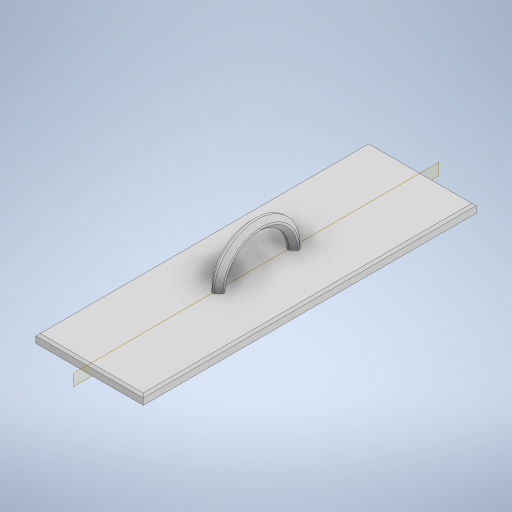
# Autodesk Inventor part: water lock
Saved by Autodesk Inventor 2023 (Build 270158000, 158)
## iProperties
Created: 2022-11-25
Part Number: water lock
Material: Generic
Document SubType Name: Sheet Metal
Designer: hp
Density: 1 g/cm^3
Sheet Metal Rule: Default_mm
Appearance: Default
Author: hp
Autodesk Inventor part; units mm, degrees
ref_plane "YZ Plane" through (0, 0, 0) normal (1, 0, 0) x (0, 1, 0)
ref_plane "XZ Plane" through (0, 0, 0) normal (0, 1, 0) x (-1, 0, 0)
ref_plane "XY Plane" through (0, 0, 0) normal (0, 0, 1) x (1, 0, 0)
sketch "Sketch1" plane through (0, 0, 0) normal (0, 1, 0) x (-1, 0, 0)
  line L0 (0, 0) -> (50, 0)
  line L1 (50, 0) -> (50, -155)
  line L2 (50, -155) -> (0, -155)
  line L3 (0, -155) -> (0, 0)
  dimension "d0" = 155
  dimension "d1" = 50
  constraints: 8 end point, 2 parallel, 1 horizontal, 1 perpendicular
  measures "d0" distance of L2.end L0.start
  measures "d1" distance of L1.end L2.end
extrude "Extrusion1" add sketch "Sketch1" along normal blind 5
sketch "Sketch2" plane through (0, 0, 0) normal (0, -1, 0) x (1, 0, 0)
  line L0 (-6, -6.5) -> (-44, -6.5)
  line L1 (-44, -6.5) -> (-44, -148.5)
  line L2 (-44, -148.5) -> (-6, -148.5)
  line L3 (-6, -148.5) -> (-6, -6.5)
  line L4 (0, 0) -> (0, -155) projected
  line L5 (0, -155) -> (-50, -155) projected
  dimension "d4" = 38
  dimension "d5" = 142
  dimension "d6" = 6
  dimension "d7" = 6.5
  constraints: 8 end point, 2 parallel, 1 horizontal, 1 perpendicular
  measures "d4" distance between parallel lines of L1 L3
  measures "d5" distance of L2.end L0.start
  measures "d6" distance between parallel lines of L4 L3
  measures "d7" distance between parallel lines of L2 L5
extrude "Extrusion2" add sketch "Sketch2" along normal blind 5
ref_plane "Work Plane1" through (-25, 0, 0) normal (1, 0, 0) x (0, 0, -1)
sketch "Sketch3" plane through (-25, 0, 0) normal (1, 0, 0) x (0, 0, -1)
  line L0 (155, 5) -> (0, 5) projected
  arc A0 (97.5, 5) -> (57.5, 5) centre (77.5, 5) ccw
  arc A1 (92.5, 5) -> (62.5, 5) centre (77.5, 5) ccw
  point P0 (0, 0)
  point P1 (73.9182, 2.8954)
  point P2 (77.5, 5)
  point P3 (77.5, 5)
  point P4 (77.5, 25)
  point P5 (77.5, 20)
  dimension "d11" = 77.5
  dimension "d12" = 0
  dimension "d13" = 20
  dimension "d14" = 20
  dimension "d15" = 20
  dimension "d16" = 5
  dimension "d17" = 5
  dimension "d18" = 5
  constraints: 6 point on circle, 4 point on line, 2 centre point, 1 midpoint
  measures "d11" distance of L0.start point (77.5, 5)
  measures "d12" distance from line of L0 point (77.5, 5)
  measures "d13" distance of A0.end point (77.5, 5)
  measures "d14" distance of A0.start point (77.5, 5)
  measures "d15" distance of point (77.5, 5) point (77.5, 25)
  measures "d16" distance of A0.end A1.end
  measures "d17" distance of A0.start A1.start
  measures "d18" distance of point (77.5, 25) point (77.5, 20)
extrude "Extrusion3" add sketch "Sketch3" along normal mid plane 5 contours L0 A1 A0
chamfer "Chamfer1" distance 2 angle 45 4 edges at (-22.5, 25, -77.5) (-27.5, 25, -77.5) (-22.5, 20, -77.5) (-27.5, 20, -77.5)
chamfer "Chamfer2" distance 1 angle 45 8 edges at (0, 5, -77.5) (-25, 5, -155) (-50, 5, -77.5) (-25, 5, 0) (-25, 0, -155) (0, 0, -77.5) (-50, 0, -77.5) (-25, 0, 0)
chamfer "Chamfer3" distance 1 angle 45 4 edges at (-25, -5, -6.5) (-44, -5, -77.5) (-6, -5, -77.5) (-25, -5, -148.5)
equation "\"BendRadius\" = Thickness"
equation "\"BendReliefWidth\" = Thickness"
equation "\"BendReliefDepth\" = 0.5 * Thickness"
equation "\"CornerReliefSize\" = 4 * Thickness"
equation "\"MinimumRemnant\" = 2 * Thickness"
equation "\"TransitionRadius\" = BendRadius"
equation "\"JacobiRadiusSize\" = BendRadius"
equation "\"GapSize\" = Thickness"
equation "\"Thickness\" = 0.5"
body "Solid1"
